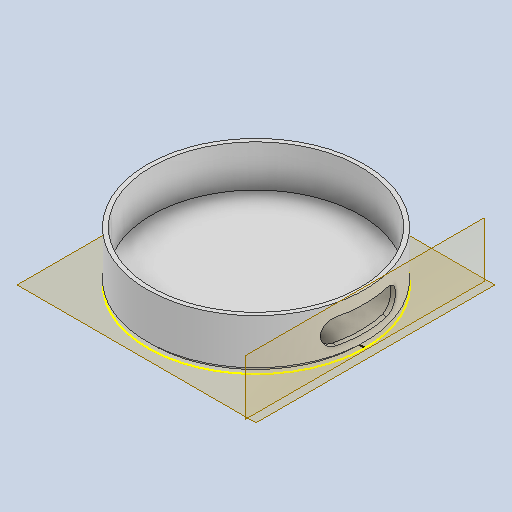
# Autodesk Inventor part: Gehaeuse_prototyp
Saved by Autodesk Inventor 2023 (Build 270158000, 158)
## iProperties
Created: 2022-06-11
Part Number: Gehaeuse_prototyp
Material: Generic
Document SubType Name: Modeling
Designer: Habib
Density: 1 g/cm^3
Appearance: Default
Author: Habib
Autodesk Inventor part; units mm, degrees
ref_plane "XY Plane" through (0, 0, 0) normal (0, 0, 1) x (1, 0, 0)
sketch "Sketch2" plane through (0, 0, 0) normal (0, 1, 0) x (-1, 0, 0)
  circle A0 centre (0, 0) radius 65
  dimension "d0" = 130
  constraints: 1 centre point, 1 coincident
  measures "d0" diameter of A0
extrude "Extrusion1" add sketch "Sketch2" along normal blind 30
sketch "Sketch3" plane through (0, 30, 0) normal (0, 1, 0) x (1, 0, 0)
  circle A0 centre (0, 0) radius 62.5
  dimension "d3" = 125
  constraints: 1 centre point, 1 coincident
  measures "d3" diameter of A0
extrude "Extrusion2" cut sketch "Sketch3" against normal blind 25
chamfer "Chamfer1" distance 3 angle 45 1 edges at (65, 0, 0)
sketch "Sketch4" plane through (0, 0, 0) normal (0, 1, 0) x (-1, 0, 0)
  line L0 (0, 0) -> (-65, 0)
  circle A0 centre (0, 0) radius 65 projected
  constraints: 2 end point, 1 horizontal, 1 horizontal alignment, 1 other
ref_plane "Work Plane1" through (65, 0, 0) normal (1, 0, 0) x (0, 1, 0)
sketch "Sketch5" plane through (65, 0, 0) normal (1, 0, 0) x (0, 1, 0)
  line L0 (15.1527, 15) -> (15.1527, -15) construction
  line L1 (7.6527, 15) -> (7.6527, -15)
  line L2 (22.6527, -15) -> (22.6527, 15)
  arc A0 (22.6527, 15) -> (7.6527, 15) centre (15.1527, 15) ccw
  arc A1 (7.6527, -15) -> (22.6527, -15) centre (15.1527, -15) ccw
  point P0 (0, 0)
  point P1 (15.1527, 0)
  dimension "d9" = 15
  dimension "d10" = 15
  constraints: 8 end point, 4 point on circle, 4 tangent, 2 centre point, 1 midpoint, 1 parallel, 1 vertical
  measures "d9" distance of point (15.153, 0) L0.end
  measures "d10" diameter of A1
extrude "Extrusion3" cut sketch "Sketch5" against normal blind 10
body "Solid1"
